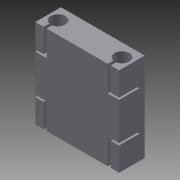
# Autodesk Inventor part: XCarriage90Body
Saved by Autodesk Inventor 2015 (Build 190159000, 159)
## iProperties
Created: 2014-10-04
Part Number: XCarriage90Body
Material: Generic
Document SubType Name: Modeling
Designer: Jack
Density: 1 g/cm^3
Appearance: Default
Author: Jack
Autodesk Inventor part; units mm, degrees
ref_plane "YZ Plane" through (0, 0, 0) normal (1, 0, 0) x (0, 1, 0)
ref_plane "XZ Plane" through (0, 0, 0) normal (0, 1, 0) x (-1, 0, 0)
ref_plane "XY Plane" through (0, 0, 0) normal (0, 0, 1) x (1, 0, 0)
sketch "Sketch1" plane through (0, 0, 0) normal (0, 0, 1) x (1, 0, 0)
  circle A0 centre (0, 0) radius 7.5 construction
  circle A1 centre (65, 0) radius 7.5 construction
  line L0 (-10, -13) -> (-10, 13)
  line L1 (-10, 13) -> (75, 13)
  line L2 (75, 13) -> (75, -13)
  line L3 (75, -13) -> (-10, -13)
  dimension "d0" = 15
  dimension "d1" = 15
  dimension "d2" = 65
  dimension "d3" = 26
  dimension "d4" = 13
  dimension "d5" = 10
  dimension "d6" = 10
  constraints: 8 end point, 3 perpendicular, 2 centre point, 1 coincident, 1 horizontal alignment, 1 vertical
  measures "d0" diameter of A0
  measures "d1" diameter of A1
  measures "d2" distance of point (0, 0) A1.centre
  measures "d3" distance of L0.start L0.end
  measures "d4" distance from line of L1 point (0, 0)
  measures "d5" distance from line of point (0, 0) L0
  measures "d6" distance from line of L2 A1.centre
extrude "Extrusion1" add sketch "Sketch1" along normal blind 90
sketch "Sketch2" plane through (0, 0, 0) normal (0, 0, -1) x (-1, 0, 0)
  line L0 (10, -13) -> (10, 13) projected
  line L1 (-75, 13) -> (-75, -13) projected
  line L2 (-75, -13) -> (10, -13) projected
  arc A0 (-63.5, -7.3485) -> (-66.5, -7.3485) centre (-65, 0) ccw
  arc A1 (1.5, -7.3485) -> (-1.5, -7.3485) centre (0, 0) ccw
  line L3 (-66.5, -7.3485) -> (-66.5, -13)
  line L4 (10, -13) -> (-75, -13) projected
  line L5 (-63.5, -7.3485) -> (-63.5, -13)
  line L6 (-1.5, -7.3485) -> (-1.5, -13)
  line L7 (1.5, -7.3485) -> (1.5, -13)
  dimension "d9" = 15
  dimension "d10" = 15
  dimension "d11" = 10
  dimension "d12" = 10
  dimension "d13" = 3
  dimension "d14" = 3
  constraints: 8 end point, 4 point on circle, 4 point on line, 3 horizontal alignment, 2 centre point, 2 parallel, 2 perpendicular, 1 coincident
  measures "d9" diameter of A0
  measures "d10" diameter of A1
  measures "d11" distance from line of L0 A1.centre
  measures "d12" distance from line of L1 A0.centre
  measures "d13" distance between parallel lines of L5 L3
  measures "d14" distance between parallel lines of L7 L6
extrude "Extrusion2" cut sketch "Sketch2" against normal blind 26
sketch "Sketch3" plane through (0, 0, 90) normal (0, 0, 1) x (1, 0, 0)
  line L0 (66.5, -13) -> (66.5, -7.3485) projected
  line L1 (63.5, -13) -> (66.5, -13) projected
  line L2 (63.5, -7.3485) -> (63.5, -13) projected
  arc A0 (66.5, -7.3485) -> (63.5, -7.3485) centre (65, 0) ccw projected
  line L3 (1.5, -13) -> (1.5, -7.3485) projected
  line L4 (-1.5, -13) -> (1.5, -13) projected
  line L5 (-1.5, -7.3485) -> (-1.5, -13) projected
  arc A1 (1.5, -7.3485) -> (-1.5, -7.3485) centre (0, 0) ccw projected
extrude "Extrusion3" cut sketch "Sketch3" against normal blind 26
sketch "Sketch4" plane through (0, 0, 64) normal (0, 0, 1) x (1, 0, 0)
  arc A0 (66.5, -7.3485) -> (63.5, -7.3485) centre (65, 0) ccw projected
  line L0 (1.5, -7.3485) -> (1.5, -13) projected
  arc A1 (1.5, -7.3485) -> (-1.5, -7.3485) centre (0, 0) ccw projected
  line L1 (-1.5, -13) -> (-1.5, -7.3485) projected
  line L2 (1.5, -13) -> (-1.5, -13) projected
  circle A2 centre (0, 0) radius 4.75
  circle A3 centre (65, 0) radius 4.75
  dimension "d19" = 9.5
  dimension "d20" = 9.5
  constraints: 2 centre point, 2 coincident
  measures "d19" diameter of A2
  measures "d20" diameter of A3
extrude "Extrusion4" cut sketch "Sketch4" against normal up to next contours A2 | A3
sketch "Sketch5" plane through (-10, -13, 0) normal (-1, 0, 0) x (0, 0, 1)
  line L0 (0, 0) -> (0, 26) projected
  line L1 (0, 0) -> (90, 0) projected
  line L2 (90, 26) -> (90, 0) projected
  line L3 (0, 26) -> (90, 26) projected
  line L4 (0, 5.6515) -> (0, 5.6515) projected
  line L5 (0, 5.6515) -> (26, 5.6515) projected
  line L6 (26, 5.6515) -> (26, 5.6515) projected
  line L7 (0, 5.6515) -> (26, 5.6515) projected
  line L8 (26, 5.6515) -> (26, 20.5) projected
  line L9 (64, 20.5) -> (64, 5.6515) projected
  line L10 (26, 20.5) -> (24, 20.5)
  line L11 (0, 20.5) -> (26, 20.5) projected
  line L12 (24, 20.5) -> (24, 0)
  line L13 (0, 0) -> (90, 0) projected
  line L14 (26, 5.6515) -> (26, 0)
  line L15 (26, 5.6515) -> (26, 0) projected
  line L16 (64, 20.5) -> (66, 20.5)
  line L17 (90, 20.5) -> (64, 20.5) projected
  line L18 (66, 20.5) -> (66, 0)
  line L19 (64, 5.6515) -> (64, 0)
  point P0 (0, 13)
  dimension "d23" = 2
  dimension "d24" = 2
  constraints: 12 end point, 4 point on line, 3 perpendicular, 1 collinear
  measures "d23" distance of L8.end L10.end
  measures "d24" distance of L9.start L16.end
extrude "Extrusion5" cut sketch "Sketch5" against normal blind 10 contours L12 L5 L14 L1 | L12 L10 L8 L5 | L19 L9 L16 L18 L1
sketch "Sketch6" plane through (75, -13, 0) normal (1, 0, 0) x (0, 0, -1)
  line L0 (0, 0) -> (-90, 0) projected
  line L1 (-66, 20.5) -> (-66, 0) projected
  line L2 (-64, 20.5) -> (-66, 20.5) projected
  line L3 (-64, 0) -> (-64, 20.5) projected
  line L4 (-26, 20.5) -> (-26, 0) projected
  line L5 (-24, 20.5) -> (-26, 20.5) projected
  line L6 (-24, 0) -> (-24, 20.5) projected
  point P0 (0, 13)
extrude "Extrusion6" cut sketch "Sketch6" against normal blind 10
body "Solid1"
